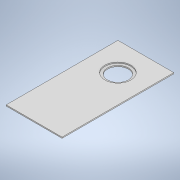
# Autodesk Inventor part: типа танк
Saved by Autodesk Inventor 2020.1 (Build 241239000, 239)
## iProperties
Created: 2022-04-04
Part Number: типа танк
Material: Типовые
Document SubType Name: Modeling
Designer: User
Density: 1 g/cm^3
Appearance: По умолчанию
Author: User
Autodesk Inventor part; units mm, degrees
ref_plane "YZ Plane" through (0, 0, 0) normal (1, 0, 0) x (0, 1, 0)
ref_plane "XZ Plane" through (0, 0, 0) normal (0, 1, 0) x (-1, 0, 0)
ref_plane "XY Plane" through (0, 0, 0) normal (0, 0, 1) x (1, 0, 0)
sketch "Эскиз1" plane through (0, 0, 0) normal (0, 1, 0) x (-1, 0, 0)
  line L0 (0, 0) -> (200, 0)
  line L1 (200, 0) -> (200, 400)
  line L2 (200, 400) -> (0, 400)
  line L3 (0, 400) -> (0, 0)
  circle A0 centre (100, 100) radius 46.5
  point P0 (100, 0)
  dimension "d0" = 200
  dimension "d1" = 400
  dimension "d2" = 100
  dimension "d3" = 93
  constraints: 8 end point, 2 parallel, 1 centre point, 1 horizontal, 1 midpoint, 1 perpendicular
  measures "d0" distance of L0.start L0.end
  measures "d1" distance of L2.end L0.start
  measures "d2" distance of point (100, 0) A0.centre
  measures "d3" diameter of A0
extrude "Выдавливание1" add sketch "Эскиз1" along normal blind 4
sketch "Эскиз2" plane through (0, 0, 0) normal (0, -1, 0) x (1, 0, 0)
  circle A0 centre (-100, 100) radius 46.5 projected
  circle A1 centre (-100, 100) radius 58.2755
  circle A2 centre (-100, 100) radius 37.4147
  point P0 (0, 0)
  constraints: 2 centre point, 2 coincident
extrude "Выдавливание2" add sketch "Эскиз2" along normal blind 4 contours A0 | A1
chamfer "Фаска1" distance 4 angle 45 1 edges at (-158.2755, 0, 100)
